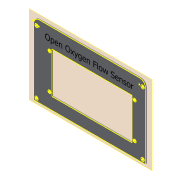
# Autodesk Inventor part: 04_Adapterplate_Display
Saved by Autodesk Inventor 2019.4 (Build 234330000, 330)
## iProperties
Created: 2021-06-04
Part Number: 04_Adapterplate_Display
Material: Generic
Document SubType Name: Modeling
Designer: diederichbenedict
Density: 1 g/cm^3
Appearance: Default
Author: diederichbenedict
Autodesk Inventor part; units mm, degrees
ref_plane "YZ Plane" through (0, 0, 0) normal (1, 0, 0) x (0, 1, 0)
ref_plane "XZ Plane" through (0, 0, 0) normal (0, 1, 0) x (-1, 0, 0)
ref_plane "XY Plane" through (0, 0, 0) normal (0, 0, 1) x (1, 0, 0)
ref_plane "Work Plane1" through (0, 0, 0) normal (0, 0, 1) x (1, 0, 0)
sketch "Sketch1" plane through (0, 0, 0) normal (0, 0, 1) x (1, 0, 0)
  circle A0 centre (2.5, -2.5) radius 1.5 projected
  circle A1 centre (95.5, -57.5) radius 1.5 projected
  circle A2 centre (95.5, -2.5) radius 1.5 projected
  circle A3 centre (2.5, -57.5) radius 1.5 projected
  line L0 (50.7939, -5.85) -> (93.3881, -5.85) projected
  line L1 (93.3881, -5.85) -> (93.3881, -53.8601) projected
  line L2 (93.3881, -53.8601) -> (4, -53.8601) projected
  line L3 (4, -53.8601) -> (4, -5.85) projected
  line L4 (4, -5.85) -> (5.9071, -5.85) projected
  line L5 (5.9071, -5.85) -> (5.9071, 0) projected
  line L6 (5.9071, 0) -> (50.7939, 0) projected
  line L7 (50.7939, 0) -> (50.7939, -5.85) projected
  line L8 (98, 3) -> (98, -60) projected
  line L9 (0, 3) -> (98, 3) projected
  line L10 (0, -60) -> (0, 3) projected
  line L11 (0, -60) -> (98, -60) projected
  line L12 (16.205, -49.4986) -> (86.205, -49.4986)
  line L13 (86.205, -49.4986) -> (86.205, -13.4986)
  line L14 (86.205, -13.4986) -> (16.205, -13.4986)
  line L15 (16.205, -13.4986) -> (16.205, -49.4986)
  line L16 (88.455, -46.9986) -> (13.955, -46.9986) construction
  line L17 (13.955, -46.9986) -> (13.955, -15.9986) construction
  line L18 (13.955, -15.9986) -> (88.455, -15.9986) construction
  line L19 (88.455, -15.9986) -> (88.455, -46.9986) construction
  line L20 (88.455, -46.9986) -> (13.955, -15.9986) construction
  line L21 (13.955, -46.9986) -> (88.455, -15.9986) construction
  circle A4 centre (13.955, -15.9986) radius 1.4
  circle A5 centre (13.955, -46.9986) radius 1.4
  circle A6 centre (88.455, -15.9986) radius 1.4 construction
  circle A7 centre (88.455, -46.9986) radius 1.4
  circle A8 centre (88.455, -15.9986) radius 1.4
  point P0 (0, 0)
  point P1 (51.205, -31.4986)
  dimension "d0" = 70
  dimension "d1" = 36
  dimension "d2" = 74.5
  dimension "d3" = 31
  dimension "d4" = 2.8
  dimension "d5" = 2.8
  dimension "d6" = 2.8
  dimension "d7" = 2.8
  constraints: 20 end point, 5 centre point, 5 coincident, 4 parallel, 2 horizontal, 2 midpoint, 2 perpendicular, 1 concentric
  measures "d0" distance between parallel lines of L13 L15
  measures "d1" distance between parallel lines of L12 L14
  measures "d2" distance of L17.end L18.end
  measures "d3" distance of L16.end L17.end
  measures "d4" diameter of A4
  measures "d5" diameter of A5
  measures "d6" diameter of A6
  measures "d7" diameter of A7
extrude "Extrusion1" add sketch "Sketch1" along normal blind 1 contours L0 L1 L2 L3 L4 L5 L6 L7 | L8 L11 L10 L9
fillet "Fillet1" radius 5 2 edges at (98, 3, 0.5) (0, 3, 0.5)
sketch "Sketch2" plane through (0, 0, 1) normal (0, 0, 1) x (1, 0, 0)
  arc A0 (5, 3) -> (0, -2) centre (5, -2) ccw projected
  line L0 (0, -2) -> (0, -60) projected
  line L1 (0, -60) -> (98, -60) projected
  line L2 (98, -60) -> (98, -2) projected
  arc A1 (98, -2) -> (93, 3) centre (93, -2) ccw projected
  line L3 (93, 3) -> (5, 3) projected
  line L4 (16.205, -49.4986) -> (16.205, -13.4986) projected
  line L5 (16.205, -13.4986) -> (86.205, -13.4986) projected
  line L6 (86.205, -13.4986) -> (86.205, -49.4986) projected
  line L7 (86.205, -49.4986) -> (16.205, -49.4986) projected
  circle A2 centre (88.455, -15.9986) radius 1.4 projected
  circle A3 centre (88.455, -46.9986) radius 1.4 projected
  circle A4 centre (13.955, -46.9986) radius 1.4 projected
  circle A5 centre (13.955, -15.9986) radius 1.4 projected
  circle A6 centre (2.5, -57.5) radius 1.5 projected
  circle A7 centre (95.5, -2.5) radius 1.5 projected
  circle A8 centre (95.5, -57.5) radius 1.5 projected
  circle A9 centre (2.5, -2.5) radius 1.5 projected
  line L8 (9.9881, -3.9779) -> (87.4866, -3.9779) construction
  line L9 (87.4866, -3.9779) -> (87.4866, -10.4067) construction
  line L10 (87.4866, -10.4067) -> (9.9881, -10.4067) construction
  line L11 (9.9881, -10.4067) -> (9.9881, -3.9779) construction
  point P0 (0, 0)
  constraints: 2 other
body "Solid1"
